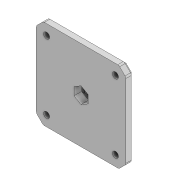
# Autodesk Inventor part: Plate_Mount
Saved by Autodesk Inventor 2020 (Build 240168000, 168)
## iProperties
Created: 2022-01-08
Part Number: Plate_Mount
Material: 一般
Document SubType Name: Modeling
Designer: ken113
Density: 1 g/cm^3
Appearance: 既定
Author: ken113
Autodesk Inventor part; units mm, degrees
ref_plane "YZ Plane" through (0, 0, 0) normal (1, 0, 0) x (0, 1, 0)
ref_plane "XZ Plane" through (0, 0, 0) normal (0, 1, 0) x (-1, 0, 0)
ref_plane "XY Plane" through (0, 0, 0) normal (0, 0, 1) x (1, 0, 0)
sketch "スケッチ1" plane through (0, 0, 0) normal (0, 0, 1) x (1, 0, 0)
  line L0 (32.5, -32.5) -> (-32.5, -32.5)
  line L1 (-32.5, -32.5) -> (-32.5, 32.5)
  line L2 (-32.5, 32.5) -> (32.5, 32.5)
  line L3 (32.5, 32.5) -> (32.5, -32.5)
  line L4 (32.5, -32.5) -> (-32.5, 32.5) construction
  line L5 (-32.5, -32.5) -> (32.5, 32.5) construction
  point P0 (0, 0)
  dimension "d0" = 65
  dimension "d1" = 65
  constraints: 12 end point, 2 midpoint, 2 parallel, 1 horizontal, 1 perpendicular
  measures "d0" distance of L1.end L2.end
  measures "d1" distance of L0.end L1.end
extrude "押し出し1" add sketch "スケッチ1" along normal blind 6
sketch "スケッチ2" plane through (0, 0, 6) normal (0, 0, 1) x (1, 0, 0)
  line L0 (0, 5.889) -> (5.1, 2.9445)
  line L1 (5.1, 2.9445) -> (5.1, -2.9445)
  line L2 (5.1, -2.9445) -> (0, -5.889)
  line L3 (0, -5.889) -> (-5.1, -2.9445)
  line L4 (-5.1, -2.9445) -> (-5.1, 2.9445)
  line L5 (-5.1, 2.9445) -> (0, 5.889)
  point P0 (0, 0)
  point P1 (0, 0)
  dimension "d4" = 10.2
  constraints: 12 end point, 1 coincident, 1 vertical alignment, 13 other
  measures "d4" distance between parallel lines of L1 L4
extrude "押し出し2" cut sketch "スケッチ2" against normal blind 5.5
sketch "スケッチ3" plane through (0, 0, 0.5) normal (0, 0, 1) x (1, 0, 0)
  circle A0 centre (0, 0) radius 3.15
  dimension "d7" = 6.3
  constraints: 1 centre point, 1 coincident
  measures "d7" diameter of A0
extrude "押し出し3" cut sketch "スケッチ3" against normal blind 5
sketch "スケッチ4" plane through (0, 0, 0) normal (0, 0, -1) x (-1, 0, 0)
  circle A0 centre (0, 0) radius 7.5
  circle A1 centre (0, 0) radius 3.15 projected
  dimension "d10" = 15
  constraints: 1 centre point, 1 coincident
  measures "d10" diameter of A0
extrude "押し出し4" add sketch "スケッチ4" along normal blind 7
chamfer "面取り1" distance 7 angle 45 1 edges at (7.5, 0, 0)
sketch "スケッチ5" plane through (0, 0, 0.5) normal (0, 0, 1) x (1, 0, 0)
  circle A0 centre (0, 0) radius 3.15 projected
  line L0 (-5.1, -2.9445) -> (-5.1, 2.9445) projected
  line L1 (0, -5.889) -> (-5.1, -2.9445) projected
  line L2 (5.1, -2.9445) -> (0, -5.889) projected
  line L3 (5.1, 2.9445) -> (5.1, -2.9445) projected
  line L4 (0, 5.889) -> (5.1, 2.9445) projected
  line L5 (-5.1, 2.9445) -> (0, 5.889) projected
  line L6 (-7.9011, 3.15) -> (7.9011, 3.15)
  line L7 (7.9011, 3.15) -> (7.9011, -3.15)
  line L8 (7.9011, -3.15) -> (-7.9011, -3.15)
  line L9 (-7.9011, -3.15) -> (-7.9011, 3.15)
  line L10 (-7.9011, 3.15) -> (7.9011, -3.15) construction
  line L11 (7.9011, 3.15) -> (-7.9011, -3.15) construction
  point P0 (4.744, 3.15)
  point P1 (0, 3.15)
  point P2 (0, -3.15)
  point P3 (4.744, -3.15)
  point P4 (-4.744, -3.15)
  point P5 (-4.744, 3.15)
  constraints: 12 end point, 2 midpoint, 2 parallel, 1 horizontal, 1 perpendicular, 1 tangent
extrude "押し出し5" cut sketch "スケッチ5" against normal blind 0.2 contours A0 L6 L4 L3 L2 L8 | A0 L8 L1 L0 L5 L6
sketch "スケッチ6" plane through (0, 0, 0.3) normal (0, 0, 1) x (1, 0, 0)
  arc A0 (0, -3.15) -> (0, 3.15) centre (0, 0) ccw projected
  line L0 (-5.1, 2.9445) -> (-4.744, 3.15) projected
  line L1 (-5.1, -2.9445) -> (-5.1, 2.9445) projected
  line L2 (-4.744, -3.15) -> (-5.1, -2.9445) projected
  line L3 (0, -3.15) -> (-4.744, -3.15) projected
  arc A1 (0, 3.15) -> (0, -3.15) centre (0, 0) ccw projected
  line L4 (-4.744, 3.15) -> (0, 3.15) projected
  line L5 (-3.15, -3.9643) -> (3.15, -3.9643)
  line L6 (3.15, -3.9643) -> (3.15, 3.9643)
  line L7 (3.15, 3.9643) -> (-3.15, 3.9643)
  line L8 (-3.15, 3.9643) -> (-3.15, -3.9643)
  line L9 (-3.15, -3.9643) -> (3.15, 3.9643) construction
  line L10 (3.15, -3.9643) -> (-3.15, 3.9643) construction
  line L11 (-4.744, 3.15) -> (4.744, 3.15) projected
  line L12 (4.744, -3.15) -> (0, -3.15) projected
  line L13 (4.744, -3.15) -> (-4.744, -3.15) projected
  line L14 (0, -5.889) -> (-4.744, -3.15) projected
  line L15 (4.744, -3.15) -> (0, -5.889) projected
  line L16 (-4.744, 3.15) -> (4.744, 3.15) projected
  line L17 (0, 5.889) -> (4.744, 3.15) projected
  line L18 (-4.744, 3.15) -> (0, 5.889) projected
  point P0 (0, -3.15)
  point P1 (0, -3.15)
  point P2 (3.15, -3.15)
  point P3 (3.15, 0)
  point P4 (3.15, 3.15)
  point P5 (0, 3.15)
  point P6 (0, 3.15)
  point P7 (-3.15, 3.15)
  point P8 (-3.15, 0)
  point P9 (-3.15, -3.15)
  constraints: 12 end point, 2 midpoint, 2 parallel, 1 horizontal, 1 perpendicular, 1 tangent
extrude "押し出し6" cut sketch "スケッチ6" against normal blind 0.2 contours L3 L8 A1 | A0 L6 L12 | A0 L11 L6 | L8 L4 A1
sketch "スケッチ7" plane through (0, 0, 0) normal (0, 0, -1) x (-1, 0, 0)
  line L0 (-25, 25) -> (25, 25)
  line L1 (25, 25) -> (25, -25)
  line L2 (25, -25) -> (-25, -25)
  line L3 (-25, -25) -> (-25, 25)
  line L4 (-25, 25) -> (25, -25) construction
  line L5 (25, 25) -> (-25, -25) construction
  point P0 (0, 0)
  dimension "d20" = 50
  dimension "d21" = 50
  constraints: 12 end point, 2 midpoint, 2 parallel, 1 horizontal, 1 perpendicular
  measures "d20" distance of L1.end L2.end
  measures "d21" distance of L0.end L1.end
hole "穴1" at (-25, 25, 0) at (25, 25, 0) at (25, -25, 0) at (-25, -25, 0) direction (0, 0, 1) diameter 4.4 end through all
sketch "スケッチ8" plane through (0, 0, 0) normal (0, 0, -1) x (-1, 0, 0)
  circle A0 centre (-25, -25) radius 2.2 projected
  circle A1 centre (25, 25) radius 2.2 projected
  circle A2 centre (-25, 25) radius 2.2 projected
  circle A3 centre (25, -25) radius 2.2 projected
  line L0 (-32.5, 32.5) -> (32.5, 32.5) projected
  line L1 (-32.5, -32.5) -> (-32.5, 32.5) projected
  line L2 (32.5, -32.5) -> (-32.5, -32.5) projected
  line L3 (32.5, 32.5) -> (32.5, -32.5) projected
  circle A4 centre (0, 0) radius 14.5 projected
  circle A5 centre (25, 25) radius 2.2 projected
  line L4 (28.2909, 25) -> (26.6454, 22.15)
  line L5 (26.6454, 22.15) -> (23.3546, 22.15)
  line L6 (23.3546, 22.15) -> (21.7091, 25)
  line L7 (21.7091, 25) -> (23.3546, 27.85)
  line L8 (23.3546, 27.85) -> (26.6454, 27.85)
  line L9 (26.6454, 27.85) -> (28.2909, 25)
  circle A6 centre (25, -25) radius 2.2 projected
  line L10 (28.2909, -25) -> (26.6454, -27.85)
  line L11 (26.6454, -27.85) -> (23.3546, -27.85)
  line L12 (23.3546, -27.85) -> (21.7091, -25)
  line L13 (21.7091, -25) -> (23.3546, -22.15)
  line L14 (23.3546, -22.15) -> (26.6454, -22.15)
  line L15 (26.6454, -22.15) -> (28.2909, -25)
  circle A7 centre (-25, -25) radius 2.2 projected
  line L16 (-21.7091, -25) -> (-23.3546, -27.85)
  line L17 (-23.3546, -27.85) -> (-26.6454, -27.85)
  line L18 (-26.6454, -27.85) -> (-28.2909, -25)
  line L19 (-28.2909, -25) -> (-26.6454, -22.15)
  line L20 (-26.6454, -22.15) -> (-23.3546, -22.15)
  line L21 (-23.3546, -22.15) -> (-21.7091, -25)
  line L22 (-21.7091, 25) -> (-23.3546, 22.15)
  line L23 (-23.3546, 22.15) -> (-26.6454, 22.15)
  line L24 (-26.6454, 22.15) -> (-28.2909, 25)
  line L25 (-28.2909, 25) -> (-26.6454, 27.85)
  line L26 (-26.6454, 27.85) -> (-23.3546, 27.85)
  line L27 (-23.3546, 27.85) -> (-21.7091, 25)
  dimension "d29" = 5.7
  dimension "d30" = 5.7
  constraints: 48 end point, 6 horizontal alignment, 4 coincident, 52 other
  measures "d29" distance between parallel lines of L5 L8
  measures "d30" distance between parallel lines of L11 L14
extrude "押し出し7" cut sketch "スケッチ8" against normal blind 2 contours L4 L5 L6 L7 L8 L9 | L10 L11 L12 L13 L14 L15 | L16 L17 L18 L19 L20 L21 | L22 L23 L24 L25 L26 L27
chamfer "面取り2" distance 5 angle 45 4 edges at (-32.5, 32.5, 3) (-32.5, -32.5, 3) (32.5, 32.5, 3) (32.5, -32.5, 3)
fillet "フィレット1" radius 2 8 edges at (32.5, 27.5, 3) (27.5, 32.5, 3) (-27.5, 32.5, 3) (-32.5, 27.5, 3) (-32.5, -27.5, 3) (-27.5, -32.5, 3) (27.5, -32.5, 3) (32.5, -27.5, 3)
chamfer "面取り3" distance 2 angle 45 16 edges at (-32.5, 0, 0) (-32.3478, -27.4369, 0) (-30, -30, 0) (-27.4369, -32.3478, 0) (0, -32.5, 0) (27.4369, -32.3478, 0) (30, -30, 0) (32.3478, -27.4369, 0) (32.5, 0, 0) (32.3478, 27.4369, 0) (30, 30, 0) (27.4369, 32.3478, 0) (0, 32.5, 0) (-27.4369, 32.3478, 0) (-30, 30, 0) (-32.3478, 27.4369, 0)
equation "\"d0\" = d1"
